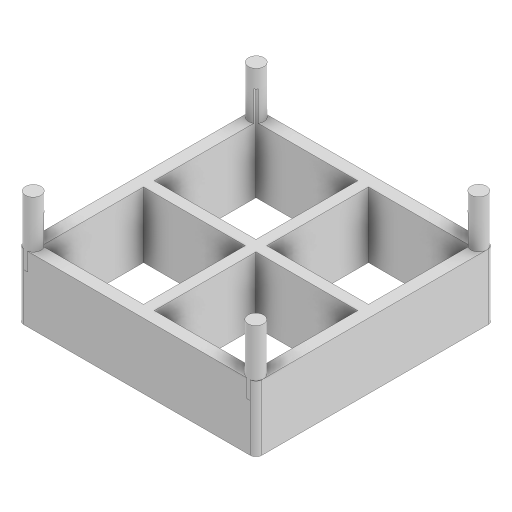
# Autodesk Inventor part: skirt
Saved by Autodesk Inventor 2023 (Build 270158000, 158)
## iProperties
Created: 2023-12-06
Part Number: skirt
Material: Generic
Document SubType Name: Modeling
Designer: ferrerx
Density: 1 g/cm^3
Appearance: Default
Author: ferrerx
Autodesk Inventor part; units mm, degrees
ref_plane "YZ Plane" through (0, 0, 0) normal (1, 0, 0) x (0, 1, 0)
ref_plane "XZ Plane" through (0, 0, 0) normal (0, 1, 0) x (-1, 0, 0)
ref_plane "XY Plane" through (0, 0, 0) normal (0, 0, 1) x (1, 0, 0)
sketch "Sketch1" plane through (0, 0, 0) normal (0, 1, 0) x (-1, 0, 0)
  line L0 (-9.35, 9.3695) -> (9.35, 9.3695) construction
  line L1 (9.35, 9.3695) -> (9.35, -9.3695) construction
  line L2 (9.35, -9.3695) -> (-9.35, -9.3695) construction
  line L3 (-9.35, -9.3695) -> (-9.35, 9.3695) construction
  line L4 (-9.35, 9.3695) -> (9.35, -9.3695) construction
  line L5 (9.35, 9.3695) -> (-9.35, -9.3695) construction
  line L6 (-10, 10) -> (10, 10)
  line L7 (10, 10) -> (10, -10)
  line L8 (10, -10) -> (-10, -10)
  line L9 (-10, -10) -> (-10, 10)
  line L10 (-10, 10) -> (10, -10) construction
  line L11 (10, 10) -> (-10, -10) construction
  point P0 (0, 0)
  dimension "d0" = 18.739
  dimension "d1" = 18.7
  dimension "d2" = 20
  dimension "d3" = 20
  constraints: 24 end point, 4 midpoint, 4 parallel, 2 horizontal, 2 perpendicular
  measures "d0" distance of L0.end L1.end
  measures "d1" distance of L1.end L2.end
  measures "d2" distance of L7.end L8.end
  measures "d3" distance of L8.end L6.start
extrude "Extrusion1" add sketch "Sketch1" along normal blind 1.5
sketch "Sketch2" plane through (0, 0, 0) normal (0, -1, 0) x (1, 0, 0)
  line L0 (-9.35, 9.3695) -> (9.35, 9.3695) construction
  line L1 (9.35, 9.3695) -> (9.35, -9.3695) construction
  line L2 (9.35, -9.3695) -> (-9.35, -9.3695) construction
  line L3 (-9.35, -9.3695) -> (-9.35, 9.3695) construction
  line L4 (-9.35, 9.3695) -> (9.35, -9.3695) construction
  line L5 (9.35, 9.3695) -> (-9.35, -9.3695) construction
  circle A0 centre (9.35, 9.3695) radius 0.65
  circle A1 centre (-9.35, 9.3695) radius 0.65
  line L6 (-10, -10) -> (-10, 10) projected
  circle A2 centre (9.35, -9.3695) radius 0.65
  circle A3 centre (-9.35, -9.3695) radius 0.65
  point P0 (0, 0)
  dimension "d6" = 1.3
  dimension "d7" = 18.739
  dimension "d8" = 18.7
  dimension "d9" = 1.3
  dimension "d11" = 1.3
  dimension "d12" = 1.3
  constraints: 12 end point, 4 centre point, 4 coincident, 2 midpoint, 2 parallel, 1 horizontal, 1 perpendicular
  measures "d6" diameter of A0
  measures "d7" distance of L0.end L1.end
  measures "d8" distance of L0.start L0.end
  measures "d9" diameter of A2
  measures "d11" diameter of A1
  measures "d12" diameter of A3
extrude "Extrusion2" add sketch "Sketch2" against normal blind 5.5
sketch "Sketch3" plane through (0, 0, 0) normal (0, -1, 0) x (1, 0, 0)
  line L0 (-10, 10) -> (10, 10) projected
  line L1 (10, -10) -> (-10, -10)
  line L2 (-10, -10) -> (-10, 10)
  line L3 (-10, 10) -> (10, 10)
  line L4 (10, 10) -> (10, -10)
  line L5 (10, -10) -> (-10, 10) construction
  line L6 (-10, -10) -> (10, 10) construction
  line L7 (9, -9) -> (-9, -9)
  line L8 (-9, -9) -> (-9, 9)
  line L9 (-9, 9) -> (9, 9)
  line L10 (9, 9) -> (9, -9)
  line L11 (9, -9) -> (-9, 9) construction
  line L12 (-9, -9) -> (9, 9) construction
  point P0 (0, 0)
  dimension "d15" = 1
  dimension "d16" = 1
  constraints: 24 end point, 4 midpoint, 4 parallel, 2 horizontal, 2 perpendicular
  measures "d15" distance between parallel lines of L0 L9
  measures "d16" distance between parallel lines of L2 L8
extrude "Extrusion3" add sketch "Sketch3" along normal blind 4
sketch "Sketch4" plane through (0, 0, 0) normal (0, -1, 0) x (1, 0, 0)
  line L0 (-9, 9) -> (-9, -9) projected
  line L1 (9, -0.45) -> (-9, -0.45)
  line L2 (-9, -0.45) -> (-9, 0.45)
  line L3 (-9, 0.45) -> (9, 0.45)
  line L4 (9, 0.45) -> (9, -0.45)
  line L5 (9, -0.45) -> (-9, 0.45) construction
  line L6 (-9, -0.45) -> (9, 0.45) construction
  line L7 (-9, -9) -> (9, -9) projected
  line L8 (0.45, 9) -> (-0.45, 9)
  line L9 (-0.45, 9) -> (-0.45, -9)
  line L10 (-0.45, -9) -> (0.45, -9)
  line L11 (0.45, -9) -> (0.45, 9)
  line L12 (0.45, 9) -> (-0.45, -9) construction
  line L13 (-0.45, 9) -> (0.45, -9) construction
  point P0 (0, 0)
  point P1 (-9, 8.8822)
  point P2 (-9, -8.8822)
  point P3 (-8.8773, -9)
  point P4 (8.8773, -9)
  point P5 (0.45, -0.45)
  point P6 (0.45, 0.45)
  point P7 (-0.45, 0.45)
  point P8 (-0.45, -0.45)
  dimension "d19" = 0.9
  dimension "d20" = 0.9
  constraints: 24 end point, 4 midpoint, 4 parallel, 2 horizontal, 2 perpendicular, 2 point on line
  measures "d19" distance between parallel lines of L11 L9
  measures "d20" distance between parallel lines of L1 L3
extrude "Extrusion4" add sketch "Sketch4" along normal blind 4 contours L3 L9 L1 L0 | L9 L8 L11 L3 | L3 L11 L1 L9 | L1 L11 L7 L9 | L3 L4 L1 L11
fillet "Fillet1" radius 0.5 4 edges at (10, -1.25, 10) (-10, -1.25, 10) (10, -1.25, -10) (-10, -1.25, -10)
sketch "Sketch5" plane through (0, 0, 0) normal (0, -1, 0) x (1, 0, 0)
  line L0 (-9, -9) -> (-0.45, -9) projected
  line L1 (-0.45, -9) -> (-0.45, -0.45) projected
  line L2 (-9, -9) -> (-0.45, -9)
  line L3 (-0.45, -9) -> (-0.45, -0.45)
  line L4 (-0.45, -0.45) -> (-9, -0.45)
  line L5 (-9, -0.45) -> (-9, -9)
  line L6 (-9, 0.45) -> (-0.45, 0.45) projected
  line L7 (-0.45, 9) -> (-9, 9) projected
  line L8 (-9, 0.45) -> (-0.45, 0.45)
  line L9 (-0.45, 0.45) -> (-0.45, 9)
  line L10 (-0.45, 9) -> (-9, 9)
  line L11 (-9, 9) -> (-9, 0.45)
  line L12 (0.45, -9) -> (9, -9) projected
  line L13 (9, -9) -> (9, -0.45) projected
  line L14 (0.45, -9) -> (9, -9)
  line L15 (9, -9) -> (9, -0.45)
  line L16 (9, -0.45) -> (0.45, -0.45)
  line L17 (0.45, -0.45) -> (0.45, -9)
  line L18 (0.45, 0.45) -> (9, 0.45) projected
  line L19 (9, 0.45) -> (9, 9) projected
  line L20 (0.45, 0.45) -> (9, 0.45)
  line L21 (9, 0.45) -> (9, 9)
  line L22 (9, 9) -> (0.45, 9)
  line L23 (0.45, 9) -> (0.45, 0.45)
  point P0 (0, 0)
  point P1 (-0.45, 0.45)
  constraints: 32 end point, 8 parallel, 4 horizontal, 4 perpendicular
extrude "Extrusion5" cut sketch "Sketch5" against normal blind 4
body "Solid1"
